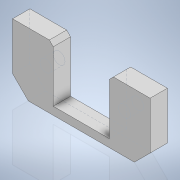
# Autodesk Inventor part: switch_stabalizer
Saved by Autodesk Inventor 2021 (Build 250183000, 183)
## iProperties
Created: 2023-07-15
Part Number: switch_stabalizer
Material: Generic
Document SubType Name: Modeling
Designer: Toby
Density: 1 g/cm^3
Appearance: Default
Author: Toby
Autodesk Inventor part; units mm, degrees
ref_plane "YZ Plane" through (0, 0, 0) normal (1, 0, 0) x (0, 1, 0)
ref_plane "XZ Plane" through (0, 0, 0) normal (0, 1, 0) x (-1, 0, 0)
ref_plane "XY Plane" through (0, 0, 0) normal (0, 0, 1) x (1, 0, 0)
sketch "Sketch1" plane through (0, 0, 0) normal (0, 0, 1) x (1, 0, 0)
  line L0 (-25.8374, 8.7301) -> (-15.4874, 8.7301)
  line L1 (-15.4874, 8.7301) -> (-15.4874, -7.3699)
  line L2 (-15.4874, -7.3699) -> (-25.8374, -7.3699)
  line L3 (-25.8374, -7.3699) -> (-25.8374, 8.7301)
  line L4 (-15.4874, -7.3699) -> (-1.1874, -7.3699)
  line L5 (-1.1874, -7.3699) -> (-1.1874, -5.3699)
  line L6 (-1.1874, -5.3699) -> (-15.4874, -5.3699)
  line L7 (-15.4874, -5.3699) -> (-15.4874, -7.3699)
  line L8 (-1.1874, -7.3699) -> (9.1626, -7.3699)
  line L9 (9.1626, -7.3699) -> (9.1626, 8.7301)
  line L10 (9.1626, 8.7301) -> (-1.1874, 8.7301)
  line L11 (-1.1874, 8.7301) -> (-1.1874, -7.3699)
  point P0 (0, 0)
  point P1 (-1.1874, -5.3699)
  point P2 (-15.4874, -5.3699)
  dimension "d0" = 35
  dimension "d1" = 14.3
  dimension "d2" = 2
  dimension "d3" = 14.1
  dimension "d4" = 10.35
  dimension "d5" = 10.35
  constraints: 24 end point, 6 parallel, 3 horizontal, 3 perpendicular, 1 point on line
  measures "d0" distance between parallel lines of L9 L3
  measures "d1" distance between parallel lines of L11 L1
  measures "d2" distance between parallel lines of L4 L6
  measures "d3" distance between parallel lines of L6 L10
  measures "d4" distance of L0.start L0.end
  measures "d5" distance of L9.end L10.end
extrude "Extrusion1" add sketch "Sketch1" along normal blind 4.4
chamfer "Chamfer1" distance 1 angle 45 2 edges at (-1.1874, 8.7301, 2.2) (-15.4874, 8.7301, 2.2)
sketch "Sketch2" plane through (0, 0, 0) normal (0, 0, -1) x (-1, 0, 0)
  line L0 (1.1874, -5.3699) -> (15.4874, -5.3699) projected
  line L1 (15.4874, -5.3699) -> (15.4874, 7.7301) projected
  line L2 (1.1874, 7.7301) -> (1.1874, -5.3699) projected
  point P0 (0, 0)
  point P1 (18.3874, 1.6301)
  point P2 (-1.6126, 1.6301)
  dimension "d12" = 7
  dimension "d13" = 7
  dimension "d14" = 20
  dimension "d15" = 2.9
  dimension "d16" = 2.8
  measures "d12" distance from line of L0 point (18.387, 1.63)
  measures "d13" distance from line of L0 point (-1.613, 1.63)
  measures "d14" distance of point (-1.613, 1.63) point (18.387, 1.63)
  measures "d15" distance from line of L1 point (18.387, 1.63)
  measures "d16" distance from line of L2 point (-1.613, 1.63)
hole "Hole1" at (-18.3874, 1.6301, 0) at (1.6126, 1.6301, 0) direction (0, 0, 1) diameter 3 depth 3.4
chamfer "Chamfer2" distance 4 angle 45 2 edges at (9.1626, -7.3699, 2.2) (-25.8374, -7.3699, 2.2)
body "Solid1"
